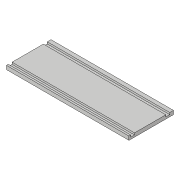
# Autodesk Inventor part: Electronics Container Part 3
Saved by Autodesk Inventor 2018.3 (Build 223284000, 284)
## iProperties
Created: 2019-03-04
Part Number: Electronics Container Part 3
Material: Generic
Document SubType Name: Modeling
Designer: aye06091
Mass: 11.5717 g
Surface Area: 95.3538 cm^2
Volume: 11.5717 cm^3
Density: 1 g/cm^3
Appearance: Default
Author: aye06091
Autodesk Inventor part; units mm, degrees
ref_plane "YZ Plane" through (0, 0, 0) normal (1, 0, 0) x (0, 1, 0)
ref_plane "XZ Plane" through (0, 0, 0) normal (0, 1, 0) x (-1, 0, 0)
ref_plane "XY Plane" through (0, 0, 0) normal (0, 0, 1) x (1, 0, 0)
sketch "Sketch1" plane through (0, 0, 0) normal (0, 1, 0) x (-1, 0, 0)
  line L0 (0, 0) -> (-104.775, 0)
  line L1 (-104.775, 0) -> (-104.775, 38.1)
  line L2 (-104.775, 38.1) -> (0, 38.1)
  line L3 (0, 38.1) -> (0, 0)
  dimension "d0" = 104.775
  dimension "d1" = 38.1
  constraints: 8 end point, 2 parallel, 1 horizontal, 1 perpendicular
  measures "d0" distance of L0.start L0.end
  measures "d1" distance of L2.end L0.start
extrude "Extrusion1" add sketch "Sketch1" along normal blind 3.175
sketch "Sketch2" plane through (0, 3.175, 0) normal (0, 1, 0) x (1, 0, 0)
  line L0 (104.775, 0) -> (0, 0) projected
  line L1 (0, 0) -> (0, -38.1) projected
  line L2 (0, -38.1) -> (104.775, -38.1) projected
  line L3 (104.775, -38.1) -> (104.775, 0) projected
  line L4 (0, -3.175) -> (104.775, -3.175)
  line L5 (104.775, -3.175) -> (104.775, -6.604)
  line L6 (104.775, -6.604) -> (0, -6.604)
  line L7 (0, -6.604) -> (0, -3.175)
  line L8 (104.775, -33.3121) -> (0, -33.3121)
  line L9 (0, -33.3121) -> (0, -36.5125)
  line L10 (0, -36.5125) -> (104.775, -36.5125)
  line L11 (104.775, -36.5125) -> (104.775, -33.3121)
  dimension "d4" = 3.429
  dimension "d5" = 3.175
  dimension "d6" = 3.2004
  dimension "d7" = 1.5875
  constraints: 16 end point, 4 parallel, 4 point on line, 2 horizontal, 2 perpendicular
  measures "d4" distance between parallel lines of L6 L4
  measures "d5" distance between parallel lines of L0 L4
  measures "d6" distance between parallel lines of L8 L10
  measures "d7" distance between parallel lines of L2 L10
extrude "Extrusion2" cut sketch "Sketch2" against normal blind 1.5875 contours L3 L6 L1 L4 | L3 L10 L1 L8
body "Solid1"
